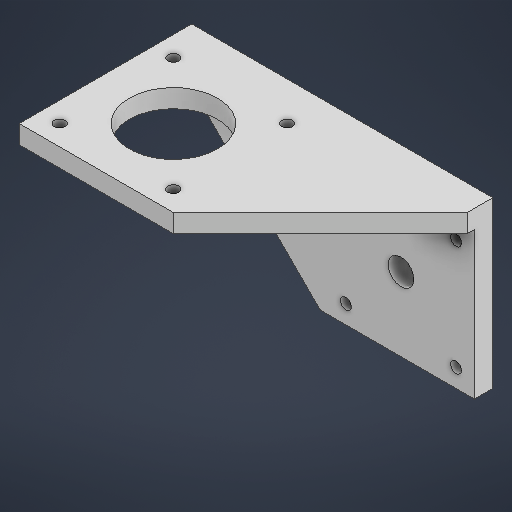
# Autodesk Inventor part: otherholderthing
Saved by Autodesk Inventor 2025.1 (Build 291241000, 241)
## iProperties
Created: 2025-02-02
Part Number: otherholderthing
Material: Generic
Document SubType Name: Modeling
Designer: jerem
Density: 1 g/cm^3
Appearance: Default
Author: jerem
## iProperties of the stored document otherholderthing_3DPrint.ipt
Created: 2025-02-02
Part Number: otherholderthing_3DPrint
Material: Generic
Document SubType Name: Modeling
Designer: jerem
Density: 1 g/cm^3
Appearance: Default
Author: jerem
Autodesk Inventor part; units mm, degrees
ref_plane "YZ Plane" through (0, 0, 0) normal (1, 0, 0) x (0, 1, 0)
ref_plane "XZ Plane" through (0, 0, 0) normal (0, 1, 0) x (-1, 0, 0)
ref_plane "XY Plane" through (0, 0, 0) normal (0, 0, 1) x (1, 0, 0)
sketch "Sketch1" plane through (0, 0, 0) normal (0, 1, 0) x (-1, 0, 0)
  line L0 (-21, 21) -> (21, 21)
  line L1 (21, 21) -> (21, -21)
  line L2 (21, -21) -> (-21, -21)
  line L3 (-21, -21) -> (-21, 21)
  line L4 (-21, 21) -> (21, -21) construction
  line L5 (21, 21) -> (-21, -21) construction
  circle A0 centre (15.5, -15.5) radius 1.5
  circle A1 centre (-15.5, -15.5) radius 1.5
  circle A2 centre (-15.5, 15.5) radius 1.5
  circle A3 centre (15.5, 15.5) radius 1.5
  line L6 (15.5, 15.5) -> (15.5, -15.5) construction
  line L7 (-15.5, -15.5) -> (15.5, -15.5) construction
  line L8 (-15.5, -15.5) -> (-15.5, 15.5) construction
  circle A4 centre (0, 0) radius 12
  line L9 (-21, 21) -> (-61, 21)
  line L10 (-61, 21) -> (-61, -21)
  line L11 (-61, -21) -> (-21, -21)
  line L12 (21, -21) -> (21, -26)
  line L13 (21, -26) -> (-61, -26)
  line L14 (-61, -26) -> (-61, -21)
  dimension "d0" = 42
  dimension "d1" = 42
  dimension "d2" = 31
  dimension "d3" = 3
  dimension "d4" = 24
  dimension "d5" = 40
  dimension "d6" = 5
  constraints: 30 end point, 7 perpendicular, 5 centre point, 4 point on line, 3 equal radius, 2 coincident, 2 horizontal, 2 midpoint, 2 parallel, 1 collinear, 1 vertical
  measures "d0" distance of L1.end L2.end
  measures "d1" distance of L0.end L1.end
  measures "d2" distance of L8.start L7.end
  measures "d3" diameter of A0
  measures "d4" diameter of A4
  measures "d5" distance between parallel lines of L3 L10
  measures "d6" distance between parallel lines of L11 L13
extrude "Extrusion1" add sketch "Sketch1" along normal blind 5
extrude "Extrusion2" add sketch "Sketch1" against normal blind 40 contours L2 L12 L13 L14 L11
sketch "Sketch2" plane through (61, 5, -26) normal (0, 0, -1) x (-1, 0, 0)
  line L0 (0, -5) -> (40, -5)
  line L1 (40, -5) -> (40, -45)
  line L2 (40, -45) -> (0, -45)
  line L3 (0, -45) -> (0, -5)
  line L4 (0, -5) -> (40, -45) construction
  line L5 (40, -5) -> (0, -45) construction
  circle A0 centre (35, -40) radius 1.5
  circle A1 centre (5, -40) radius 1.5
  circle A2 centre (5, -10) radius 1.5
  circle A3 centre (35, -10) radius 1.5
  line L6 (35, -10) -> (35, -40) construction
  line L7 (5, -40) -> (35, -40) construction
  line L8 (5, -40) -> (5, -10) construction
  circle A4 centre (20, -25) radius 3.5
  point P0 (61, -5)
  dimension "d11" = 40
  dimension "d12" = 40
  dimension "d13" = 30
  dimension "d14" = 3
  dimension "d15" = 7
  constraints: 18 end point, 5 centre point, 4 perpendicular, 4 point on line, 3 equal radius, 2 coincident, 2 midpoint, 2 parallel, 1 horizontal
  measures "d11" distance of L1.end L2.end
  measures "d12" distance of L0.end L1.end
  measures "d13" distance of L8.start L7.end
  measures "d14" diameter of A0
  measures "d15" diameter of A4
extrude "Extrusion3" cut sketch "Sketch2" against normal through all contours A0 | A1 | A2 | A3 | A4
chamfer "Chamfer1" distance 40 angle 45 1 edges at (61, 2.5, 21)
chamfer "Chamfer2" distance 40 angle 45 1 edges at (-21, -40, -23.5)
body "Solid1"
